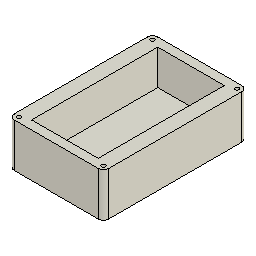
BATTERY HOLDER V1 v19 (Autodesk Fusion 360 design; units mm, degrees)
Autodesk Fusion 360 part; units mm, degrees
note: some values were not read from the file. Set by a fixed rule: which sketch regions a step uses.
sketch "Sketch1" plane through (0, 0, 0) normal (0, 0, 1) x (1, 0, 0)
  line L0 (-20, 34) -> (20, 34)
  line L1 (20, 34) -> (20, -34)
  line L2 (20, -34) -> (-20, -34)
  line L3 (-20, -34) -> (-20, 34)
  line L4 (-20, 34) -> (20, -34) construction
  line L5 (20, 34) -> (-20, -34) construction
  line L6 (27, 41) -> (27, -41)
  line L7 (27, -41) -> (-27, -41)
  line L8 (-27, -41) -> (-27, 41)
  line L9 (-27, 41) -> (27, 41)
  line L10 (0, -41) -> (0, 41)
  line L11 (27, 0) -> (-27, 0)
  line L12 (-27, -41) -> (-24.1716, -38.1716)
  line L13 (-27, -41) -> (-18.25, -41) construction
  circle A0 centre (-24.1716, -38.1716) radius 1.115
  line L14 (27, -41) -> (24.1716, -38.1716)
  circle A1 centre (24.1716, -38.1716) radius 1.115
  circle A2 centre (-24.1716, 38.1716) radius 1.115
  line L15 (-27, 41) -> (-24.1716, 38.1716)
  circle A3 centre (24.1716, 38.1716) radius 1.115
  line L16 (27, 41) -> (24.1716, 38.1716)
  circle A4 centre (-24.1716, -38.1716) radius 2
  circle A5 centre (24.1716, -38.1716) radius 2
  circle A6 centre (-24.1716, 38.1716) radius 2
  circle A7 centre (24.1716, 38.1716) radius 2
  line L17 (17.25, -24.75) -> (-17.25, -24.75)
  line L18 (-17.25, -24.75) -> (-17.25, 24.75)
  line L19 (-17.25, 24.75) -> (17.25, 24.75)
  line L20 (17.25, 24.75) -> (17.25, -24.75)
  line L21 (17.25, -24.75) -> (-17.25, 24.75) construction
  line L22 (-17.25, -24.75) -> (17.25, 24.75) construction
  line L23 (0, 24.75) -> (0, 41)
  dimension "d1" = 40
  dimension "d2" = 68
  dimension "d3" = -7
  dimension "d4" = 4
  dimension "d5" = 45
  dimension "d6" = 2.23
  dimension "d7" = 4
  dimension "d25" = 34.5
  dimension "d26" = 49.5
  dimension "d27" = 54
  dimension "d28" = 82
  constraint horizontal L0
  constraint perpendicular L0 L1
  constraint parallel L0 L2
  constraint parallel L1 L3
  constraint coincident L4 origin
  constraint coincident L5 origin
  constraint midpoint L7 L10.start
  constraint midpoint L9 L10.end
  constraint midpoint L6 L11.start
  constraint midpoint L8 L11.end
  constraint horizontal L13
  constraint coincident L12.end A0.centre
  constraint symmetric L7.end L10 L6.end
  constraint symmetric L10 L12.end L14.end
  constraint symmetric L10 A0 A1
  constraint symmetric L7.end L11 L8.end
  constraint symmetric L11 L12.end A2.centre
  constraint symmetric L11 A0 A2
  constraint symmetric L11 L6.end L6.start
  constraint symmetric L11 L14.end A3.centre
  constraint symmetric L11 A1 A3
  constraint concentric A0 A4
  constraint symmetric L10 A4 A5
  constraint symmetric L11 A4 A6
  constraint symmetric L11 A5 A7
  constraint horizontal L17
  constraint perpendicular L17 L18
  constraint parallel L17 L19
  constraint parallel L18 L20
  constraint coincident L21 origin
  constraint coincident L22 origin
  constraint midpoint L19 L23.start
  measures "d1" distance of L1.end L2.end
  measures "d2" distance of L0.end L1.end
  measures "d4" distance of L7.end L12.end
  measures "d5" angle of L12 L13
  measures "d6" diameter of A0
  measures "d7" diameter of A4
  measures "d25" distance of L18.end L19.end
  measures "d26" distance of L17.end L18.end
  measures "d27" distance of L6.end L7.end
  measures "d28" distance of L6.start L6.end
extrude "Extrude1" add sketch "Sketch1" along normal blind 20 contours A4 | A5 | A6 | A7 makes body 1 at (23.2592, -39.9513, 13.3333) makes body 2 at (-22.1815, 38.3707, 13.3333) makes body 3 at (-22.1815, -37.9724, 13.3333) makes body 4 at (26.1616, 38.3707, 13.3333)
extrude "Extrude2" add sketch "Sketch1" against normal blind 5 separate body contours L0 L3 L8 L9 L10 L11 L23 | L0 L3 L10 L11 L18 L19 L23 | L0 L1 L6 L9 L10 L11 L23 | L0 L1 L10 L11 L19 L20 L23 | L2 L3 L10 L11 L17 L18 | L2 L3 L7 L8 L10 L11 | L10 L11 L19 L20 | L10 L11 L18 L19 | L10 L11 L17 L18 | L1 L2 L6 L7 L10 L11 | L1 L2 L10 L11 L17 L20 | L10 L11 L17 L20 makes body 5
extrude "Extrude3" add sketch "Sketch1" against normal blind 5 contours A0 | A1 | A2 | A3 | A5 | A6 | A7 bodies 1 3 2 4 5
extrude "Extrude4" add sketch "Sketch1" along normal blind 20 contours L0 L3 L8 L9 L10 L11 L23 | L0 L1 L6 L9 L10 L11 L23 | L2 L3 L7 L8 L10 L11 | L1 L2 L6 L7 L10 L11 bodies 1 3
extrude "Extrude5" cut 1 faces at (-6.6667, 34, 6.6667) along direction (0, 1, 0) blind 1 on bodies 1 bodies 1
extrude "Extrude6" cut 1 faces at (-6.6667, 35, 6.6667) along direction (0, 1, 0) blind 1 on bodies 1 bodies 1
extrude "Extrude7" cut 1 faces at (6.6667, -34, 6.6667) along direction (0, -1, 0) blind 2 on bodies 1 bodies 1
extrude "Extrude8" cut sketch "Sketch1" against normal blind 100 contours A0 | A1 | A2 | A3 bodies 1
sketch "Sketch2" plane through (0, 0, -5) normal (0, 0, -1) x (1, 0, 0)
  circle A0 centre (-24.1716, -38.1716) radius 1.115
  circle A1 centre (24.1716, 38.1716) radius 1.115
  circle A2 centre (24.1716, -38.1716) radius 1.115
  circle A3 centre (-24.1716, 38.1716) radius 2
  line L0 (-27, 41) -> (-27, -41)
  line L1 (-27, -41) -> (27, -41)
  line L2 (27, -41) -> (27, 41)
  line L3 (27, 41) -> (-27, 41)
  circle A4 centre (24.1716, 38.1716) radius 2
  circle A5 centre (-24.1716, 38.1716) radius 2
  circle A6 centre (24.1716, -38.1716) radius 2
  circle A7 centre (-24.1716, -38.1716) radius 2
  dimension "d29" = 4
  dimension "d30" = 4
  dimension "d31" = 4
  dimension "d32" = 4
  constraint concentric A1 A4
  constraint concentric A3 A5
  constraint concentric A2 A6
  constraint concentric A0 A7
  measures "d29" diameter of A4
  measures "d30" diameter of A5
  measures "d31" diameter of A6
  measures "d32" diameter of A7
extrude "Extrude9" cut sketch "Sketch2" against normal blind 20 contours A3 A5 | A4 | A6 | A7 bodies 1
sketch "Sketch3" plane through (0, 41, 0) normal (0, 1, 0) x (-1, 0, 0)
  line L0 (-27, 20) -> (-27, -5)
  line L1 (-27, -5) -> (27, -5)
  line L2 (27, -5) -> (27, 20)
  line L3 (27, 20) -> (-27, 20)
  line L4 (0, -5) -> (0, 20)
  line L5 (5, 6.5) -> (-5, 6.5)
  line L6 (-5, 6.5) -> (-5, 13.5)
  line L7 (-5, 13.5) -> (5, 13.5)
  line L8 (5, 13.5) -> (5, 6.5)
  line L9 (5, 6.5) -> (-5, 13.5) construction
  line L10 (-5, 6.5) -> (5, 13.5) construction
  point P0 (0, 10)
  dimension "d35" = 10
  dimension "d36" = 7
  constraint midpoint L1 L4.start
  constraint midpoint L3 L4.end
  constraint horizontal L5
  constraint perpendicular L5 L6
  constraint parallel L5 L7
  constraint parallel L6 L8
  constraint coincident L9 P0
  constraint coincident L10 P0
  constraint coincident L4 P0
  measures "d35" distance of L6.end L7.end
  measures "d36" distance of L5.end L6.end
extrude "Extrude10" cut sketch "Sketch3" against normal blind 16 contours L4 L5 L7 L8 | L4 L5 L6 L7 bodies 1
fillet "Fillet1" radius 4 4 edges at (-27, 41, 7.5) (27, 41, 7.5) (27, -41, 7.5) (-27, -41, 7.5) on bodies 1
extrude "Extrude21" add 1 faces at (-5, 37.6667, 11.1667) along direction (1, 0, 0) blind 10 on bodies 1 bodies 1
extrude "Extrude22" add 1 faces at (-20, 12, 13.3333) along direction (1, 0, 0) blind 1 on bodies 1 bodies 1
extrude "Extrude23" add 1 faces at (20, -12, 13.3333) along direction (-1, 0, 0) blind 1 on bodies 1 bodies 1
delete_face "DeleteFace1" 1 faces at (23.1903, -40.9955, 11.6667) on bodies 1
delete_face "DeleteFace2" 1 faces at (26.9955, 37.1903, 11.6667) on bodies 1
delete_face "DeleteFace3" 1 faces at (-23.3802, -40.9819, 3.3333) on bodies 1
delete_face "DeleteFace4" 1 faces at (-26.9955, 37.1903, 3.3333) on bodies 1
fillet "Fillet5" radius 3 4 edges at (-27, 41, 7.5) (-27, -41, 7.5) (27, -41, 7.5) (27, 41, 7.5) on bodies 1
extrude "Extrude11" [suppressed]
extrude "Extrude12" [suppressed]
extrude "Extrude13" [suppressed]
extrude "Extrude14" [suppressed]
extrude "Extrude15" [suppressed]
extrude "Extrude16" [suppressed]
extrude "Extrude17" [suppressed]
extrude "Extrude18" [suppressed]
fillet "Fillet2" [suppressed]
sketch "Sketch4" plane through (0, 0, -5) normal (0, 0, -1) x (1, 0, 0)
  arc A0 (-23, 41) -> (-27, 37) centre (-23, 37) ccw
  line L0 (-27, 37) -> (-30, 37)
  line L1 (-30, 37) -> (-30, -37)
  line L2 (-30, -37) -> (-27, -37)
  arc A1 (-27, -37) -> (-23, -41) centre (-23, -37) ccw
  line L3 (-23, -41) -> (-23, -44)
  line L4 (-23, -44) -> (23, -44)
  line L5 (23, -44) -> (23, -41)
  arc A2 (23, -41) -> (27, -37) centre (23, -37) ccw
  line L6 (27, -37) -> (30, -37)
  line L7 (30, -37) -> (30, 37)
  line L8 (30, 37) -> (27, 37)
  arc A3 (27, 37) -> (23, 41) centre (23, 37) ccw
  line L9 (23, 41) -> (23, 44)
  line L10 (23, 44) -> (-23, 44)
  line L11 (-23, 44) -> (-23, 41)
  circle A4 centre (24.1716, -38.1716) radius 2
  circle A5 centre (24.1716, 38.1716) radius 2
  circle A6 centre (-24.1716, -38.1716) radius 2
  circle A7 centre (-24.1716, 38.1716) radius 2
  line L12 (-30, -44) -> (30, -44)
  line L13 (30, -44) -> (30, 44)
  line L14 (30, 44) -> (-30, 44)
  line L15 (-30, 44) -> (-30, -44)
  constraint horizontal L12
  constraint vertical L13
  constraint horizontal L14
  constraint vertical L15
extrude "Extrude19" [suppressed]
fillet "Fillet3" [suppressed]
fillet "Fillet4" [suppressed]
sketch "Sketch5" plane through (0, 0, -5) normal (0, 0, -1) x (1, 0, 0)
  arc A0 (20, -44) -> (30, -34) centre (20, -34) ccw
  line L0 (30, -34) -> (30, 34)
  arc A1 (30, 34) -> (20, 44) centre (20, 34) ccw
  line L1 (20, 44) -> (-20, 44)
  arc A2 (-20, 44) -> (-30, 34) centre (-20, 34) ccw
  line L2 (-30, 34) -> (-30, -34)
  arc A3 (-30, -34) -> (-20, -44) centre (-20, -34) ccw
  line L3 (-20, -44) -> (20, -44)
  circle A4 centre (24.1716, -38.1716) radius 2
  circle A5 centre (24.1716, 38.1716) radius 2
  circle A6 centre (-24.1716, -38.1716) radius 2
  circle A7 centre (-24.1716, 38.1716) radius 2
  line L4 (30, -44) -> (30, 43.7522) construction
  line L5 (30, 43.7522) -> (-29.9804, 43.7522) construction
  line L6 (-29.9804, 43.7522) -> (-29.9804, -44) construction
  line L7 (-29.9804, -44) -> (30, -44) construction
  dimension "d65" = 7
extrude "Extrude20" [suppressed]
equation "d66 = 'made by  Parth Dhiman '"
